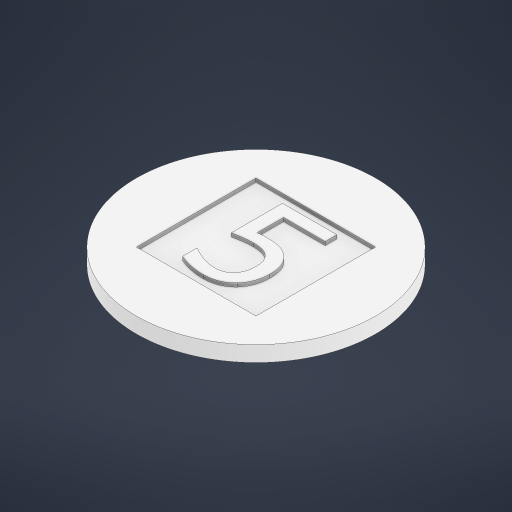
# Autodesk Inventor part: TopMarker1
Saved by Autodesk Inventor 2023.2 (Build 272271030, 271C)
## iProperties
Created: 2023-03-04
Part Number: TopMarker1
Material: Generic
Document SubType Name: Modeling
Designer: Elias Braun
Density: 1 g/cm^3
Appearance: Default
Author: Elias Braun
Autodesk Inventor part; units mm, degrees
ref_plane "YZ Plane" through (0, 0, 0) normal (1, 0, 0) x (0, 1, 0)
ref_plane "XZ Plane" through (0, 0, 0) normal (0, 1, 0) x (-1, 0, 0)
ref_plane "XY Plane" through (0, 0, 0) normal (0, 0, 1) x (1, 0, 0)
sketch "Sketch1" plane through (0, 0, 0) normal (0, 1, 0) x (-1, 0, 0)
  circle A0 centre (0, 0) radius 20
  dimension "d0" = 40
  constraints: 1 centre point, 1 coincident
  measures "d0" diameter of A0
extrude "Extrusion1" add sketch "Sketch1" along normal blind 2.6
sketch "Sketch2" plane through (0, 2.6, 0) normal (0, 1, 0) x (1, 0, 0)
  line L0 (10, -10) -> (-10, -10)
  line L1 (-10, -10) -> (-10, 10)
  line L2 (-10, 10) -> (10, 10)
  line L3 (10, 10) -> (10, -10)
  line L4 (10, -10) -> (-10, 10) construction
  line L5 (-10, -10) -> (10, 10) construction
  point P0 (0, 0)
  dimension "d3" = 20
  dimension "d4" = 20
  constraints: 12 end point, 2 midpoint, 2 parallel, 1 horizontal, 1 perpendicular
  measures "d3" distance of L0.start L0.end
  measures "d4" distance of L0.end L1.end
extrude "Extrusion2" cut sketch "Sketch2" against normal blind 0.6
sketch "Sketch4" plane through (0, 2, 0) normal (0, 1, 0) x (1, 0, 0)
  line L0 (-6.192, 8.5476) -> (6.2647, 8.5476) construction
  line L1 (6.2647, 8.5476) -> (6.2647, -8.4022) construction
  line L2 (6.2647, -8.4022) -> (-6.192, -8.4022) construction
  line L3 (-6.192, -8.4022) -> (-6.192, 8.5476) construction
  spline S0 degree 2 poles (5.0809, -2.7792) (5.0809, -3.9764) (4.3141, -6.0211) (3.6146, -6.7745) knots 0 0 0 1 2 2 2
  spline S1 degree 2 poles (3.6146, -6.7745) (2.9151, -7.5278) (0.83, -8.4022) (-0.4614, -8.4022) knots 0 0 0 1 2 2 2
  spline S2 degree 2 poles (-0.4614, -8.4022) (-1.6452, -8.4022) (-3.9589, -7.8775) (-4.8064, -7.4605) knots 0 0 0 1 2 2 2
  line L4 (-4.8064, -7.4605) -> (-4.8064, -5.1064)
  line L5 (-4.8064, -5.1064) -> (-4.645, -5.1064)
  spline S3 degree 2 poles (-4.645, -5.1064) (-4.3894, -5.2947) (-3.4343, -5.779) (-2.8559, -5.9942) knots 0 0 0 1 2 2 2
  spline S4 degree 2 poles (-2.8559, -5.9942) (-2.1967, -6.2229) (-1.1071, -6.4785) (-0.421, -6.4785) knots 0 0 0 1 2 2 2
  spline S5 degree 2 poles (-0.421, -6.4785) (0.2516, -6.4785) (1.5161, -5.9942) (1.9735, -5.4696) knots 0 0 0 1 2 2 2
  spline S6 degree 2 poles (1.9735, -5.4696) (2.3905, -4.9719) (2.821, -3.6536) (2.821, -2.7657) knots 0 0 0 1 2 2 2
  spline S7 degree 2 poles (2.821, -2.7657) (2.821, -1.8779) (2.3367, -0.7479) (1.8793, -0.3712) knots 0 0 0 1 2 2 2
  spline S8 degree 2 poles (1.8793, -0.3712) (1.4085, 0.0458) (0.0094, 0.3956) (-0.838, 0.3956) knots 0 0 0 1 2 2 2
  spline S9 degree 2 poles (-0.838, 0.3956) (-1.7528, 0.3956) (-3.5688, 0.1131) (-4.1204, -0.008) knots 0 0 0 1 2 2 2
  line L6 (-4.1204, -0.008) -> (-4.1204, 8.5476)
  line L7 (-4.1204, 8.5476) -> (4.9868, 8.5476)
  line L8 (4.9868, 8.5476) -> (4.9868, 6.597)
  line L9 (4.9868, 6.597) -> (-1.9815, 6.597)
  line L10 (-1.9815, 6.597) -> (-1.9815, 2.1712)
  spline S10 degree 2 poles (-1.9815, 2.1712) (-1.5779, 2.2251) (-0.7977, 2.2654) (-0.4748, 2.2654) knots 0 0 0 1 2 2 2
  spline S11 degree 2 poles (-0.4748, 2.2654) (0.8031, 2.2654) (2.5654, 1.8484) (3.3725, 1.2296) knots 0 0 0 1 2 2 2
  spline S12 degree 2 poles (3.3725, 1.2296) (4.1931, 0.6108) (5.0809, -1.2725) (5.0809, -2.7792) knots 0 0 0 1 2 2 2
  constraints: 2 other
extrude "Extrusion4" add sketch "Sketch4" along normal blind 0.6
body "Solid1"
